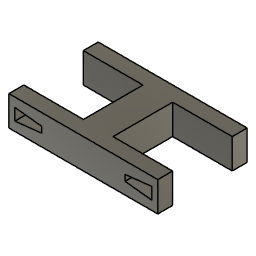
middle part (Autodesk Fusion 360 design; units mm, degrees)
Autodesk Fusion 360 part; units mm, degrees
sketch "Sketch1" plane through (0, 0, 0) normal (0, 0, 1) x (1, 0, 0)
  line L0 (0, 0) -> (50, 0)
  line L1 (50, 29.9983) -> (0, 29.9983)
  line L2 (0, 5) -> (20.0173, 5)
  line L3 (20.0173, 5) -> (20.0173, 25)
  line L4 (20.0173, 25) -> (0, 25)
  line L5 (50, 25) -> (29.9868, 25)
  line L6 (29.9868, 25) -> (29.9868, 4.9812)
  line L7 (29.9868, 4.9812) -> (50, 4.9812)
  line L8 (0, 29.9983) -> (0, 25)
  line L9 (0, 5) -> (0, 0)
  line L10 (50, 0) -> (50, 4.9812)
  line L11 (50, 25) -> (50, 29.9983)
  constraint horizontal L0
  constraint vertical L10
  constraint horizontal L1
  constraint vertical L8
  constraint coincident L0.start L9.end
  constraint horizontal L2
  constraint vertical L3
  constraint horizontal L4
  constraint coincident L2.start L8
  constraint horizontal L5
  constraint vertical L6
  constraint horizontal L7
  constraint coincident L5.start L10
  constraint collinear L8 L9
  constraint collinear L10 L11
sketch "Sketch4" plane through (0, 0, 0) normal (0, 0, 1) x (1, 0, 0)
extrude "Extrude2" add sketch "Sketch1" along normal blind 10
sketch "Sketch5" plane through (0, 0, 0) normal (0, 1, 0) x (1, 0, 0)
sketch "Sketch6" plane through (0, 0, 0) normal (0, 1, 0) x (1, 0, 0)
  line L0 (2, -7) -> (10.9982, -6.004)
  line L1 (10.9982, -6.004) -> (10.9982, -4.0183)
  line L2 (10.9982, -4.0183) -> (2, -3)
  line L3 (2, -3) -> (2, -7)
  line L4 (48, -3) -> (39, -4)
  line L5 (39, -4) -> (39, -6.004)
  line L6 (39, -6.004) -> (48, -7)
  line L7 (48, -7) -> (48, -3)
  constraint parallel L1 L3
  constraint parallel L1 L5
  constraint parallel L5 L7
extrude "Extrude3" cut sketch "Sketch6" along normal blind 6 contours L4 L5 L6 L7
sketch "Sketch7" plane through (0, 0, 0) normal (0, 1, 0) x (1, 0, 0)
  line L0 (2, -3) -> (11, -4)
  line L1 (11, -4) -> (11, -6)
  line L2 (2, -7) -> (2, -3)
  line L3 (2, -7) -> (11, -6)
  constraint vertical L1
  constraint vertical L2
extrude "Extrude4" cut sketch "Sketch7" along normal blind 6
extrude "Extrude1" [suppressed]
other "Form1"
sketch "Sketch2" plane through (0, 0, 0) normal (0, 0, 1) x (1, 0, 0)
sketch "Sketch3" plane through (0, 0, 0) normal (0, 0, 1) x (1, 0, 0)
